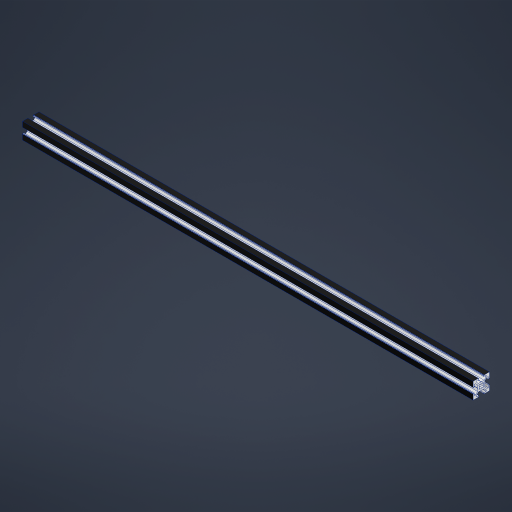
# Autodesk Inventor part: 20mm Extrusion 500mm
Saved by Autodesk Inventor 2024.2 (Build 282272000, 272)
## iProperties
Created: 2024-10-04
Part Number: 20mm Extrusion 500mm
Material: Aluminum 6061
Document SubType Name: Modeling
Designer: jerem
Density: 2.7 g/cm^3
Appearance: Aluminum - Flat
Author: jerem
Autodesk Inventor part; units mm, degrees
ref_plane "YZ Plane" through (0, 0, 0) normal (1, 0, 0) x (0, 1, 0)
ref_plane "XZ Plane" through (0, 0, 0) normal (0, 1, 0) x (-1, 0, 0)
ref_plane "XY Plane" through (0, 0, 0) normal (0, 0, 1) x (1, 0, 0)
sketch "Sketch1" plane through (0, 0, 0) normal (1, 0, 0) x (0, 1, 0)
  line L0 (-10, -10) -> (10, 10) construction
  line L1 (10, 10) -> (10, 3.5)
  line L2 (10, 3.5) -> (9.5, 3.5)
  line L3 (9.5, 3.5) -> (9.5, 3)
  line L4 (9.5, 3) -> (8.5, 3)
  line L5 (8.5, 3) -> (8.5, 5.95)
  line L6 (8.5, 5.95) -> (7.0107, 5.95)
  line L7 (7.0107, 5.95) -> (4.5, 3.4393)
  line L8 (4.5, 3.4393) -> (4.5, 0.1525)
  line L9 (2.4501, 2.4501) -> (3.0123, 1.888)
  line L10 (3.0123, 1.888) -> (2.4163, 1.292)
  arc A0 (2.74, 0) -> (2.4163, 1.292) centre (0, 0) ccw
  arc A1 (4.5, 0.1525) -> (4.3475, 0) centre (4.5, 0) ccw
  line L11 (10, 10) -> (2.4501, 2.4501)
  line L12 (4.3475, 0) -> (2.74, 0)
  line L13 (0, 0) -> (2.74, 0) construction
  line L14 (10, 10) -> (3.5, 10)
  line L15 (3.5, 10) -> (3.5, 9.5)
  line L16 (3.5, 9.5) -> (3, 9.5)
  line L17 (3, 9.5) -> (3, 8.5)
  line L18 (3, 8.5) -> (5.95, 8.5)
  line L19 (5.95, 8.5) -> (5.95, 7.0107)
  line L20 (5.95, 7.0107) -> (3.4393, 4.5)
  line L21 (3.4393, 4.5) -> (0.1525, 4.5)
  line L22 (2.4501, 2.4501) -> (1.888, 3.0123)
  line L23 (1.888, 3.0123) -> (1.292, 2.4163)
  arc A2 (1.292, 2.4163) -> (0, 2.74) centre (0, 0) ccw
  arc A3 (0, 4.3475) -> (0.1525, 4.5) centre (0, 4.5) ccw
  line L24 (0, 4.3475) -> (0, 2.74)
  line L25 (0, 0) -> (0, 2.74) construction
  line L26 (-8.5, 5.95) -> (-7.0107, 5.95)
  line L27 (-10, 3.5) -> (-9.5, 3.5)
  line L28 (-8.5, 3) -> (-8.5, 5.95)
  line L29 (-9.5, 3.5) -> (-9.5, 3)
  line L30 (-9.5, 3) -> (-8.5, 3)
  line L31 (-5.95, 8.5) -> (-5.95, 7.0107)
  line L32 (-7.0107, 5.95) -> (-4.5, 3.4393)
  line L33 (-5.95, 7.0107) -> (-3.4393, 4.5)
  line L34 (-10, 10) -> (-10, 3.5)
  line L35 (-10, 10) -> (-3.5, 10)
  line L36 (-10, 10) -> (-2.4501, 2.4501)
  line L37 (-3, 8.5) -> (-5.95, 8.5)
  line L38 (-3, 9.5) -> (-3, 8.5)
  line L39 (-3.5, 10) -> (-3.5, 9.5)
  line L40 (-3.5, 9.5) -> (-3, 9.5)
  line L41 (-3.4393, 4.5) -> (-0.1525, 4.5)
  line L42 (-2.4501, 2.4501) -> (-1.888, 3.0123)
  line L43 (-1.888, 3.0123) -> (-1.292, 2.4163)
  arc A4 (0, 2.74) -> (-1.292, 2.4163) centre (0, 0) ccw
  arc A5 (-0.1525, 4.5) -> (0, 4.3475) centre (0, 4.5) ccw
  line L44 (-2.4501, 2.4501) -> (-3.0123, 1.888)
  line L45 (-4.5, 3.4393) -> (-4.5, 0.1525)
  arc A6 (-4.3475, 0) -> (-4.5, 0.1525) centre (-4.5, 0) ccw
  line L46 (0, 4.3475) -> (0, 2.74)
  line L47 (-4.3475, 0) -> (-2.74, 0)
  arc A7 (-2.4163, 1.292) -> (-2.74, 0) centre (0, 0) ccw
  line L48 (0, 0) -> (0, 2.74) construction
  line L49 (-3.0123, 1.888) -> (-2.4163, 1.292)
  line L50 (-5.95, -8.5) -> (-5.95, -7.0107)
  line L51 (-3.5, -10) -> (-3.5, -9.5)
  line L52 (-3, -8.5) -> (-5.95, -8.5)
  line L53 (-3.5, -9.5) -> (-3, -9.5)
  line L54 (-3, -9.5) -> (-3, -8.5)
  line L55 (-8.5, -5.95) -> (-7.0107, -5.95)
  line L56 (-5.95, -7.0107) -> (-3.4393, -4.5)
  line L57 (-7.0107, -5.95) -> (-4.5, -3.4393)
  line L58 (-10, -10) -> (-3.5, -10)
  line L59 (-10, -10) -> (-10, -3.5)
  line L60 (-10, -10) -> (-2.4501, -2.4501)
  line L61 (-8.5, -3) -> (-8.5, -5.95)
  line L62 (-9.5, -3) -> (-8.5, -3)
  line L63 (-10, -3.5) -> (-9.5, -3.5)
  line L64 (-9.5, -3.5) -> (-9.5, -3)
  line L65 (-4.5, -3.4393) -> (-4.5, -0.1525)
  line L66 (-2.4501, -2.4501) -> (-3.0123, -1.888)
  line L67 (-3.0123, -1.888) -> (-2.4163, -1.292)
  arc A8 (-2.74, 0) -> (-2.4163, -1.292) centre (0, 0) ccw
  arc A9 (-4.5, -0.1525) -> (-4.3475, 0) centre (-4.5, 0) ccw
  line L68 (-2.4501, -2.4501) -> (-1.888, -3.0123)
  line L69 (-3.4393, -4.5) -> (-0.1525, -4.5)
  arc A10 (0, -4.3475) -> (-0.1525, -4.5) centre (0, -4.5) ccw
  line L70 (-4.3475, 0) -> (-2.74, 0)
  line L71 (0, -4.3475) -> (0, -2.74)
  arc A11 (-1.292, -2.4163) -> (0, -2.74) centre (0, 0) ccw
  line L72 (0, 0) -> (-2.74, 0) construction
  line L73 (-1.888, -3.0123) -> (-1.292, -2.4163)
  line L74 (8.5, -5.95) -> (7.0107, -5.95)
  line L75 (10, -3.5) -> (9.5, -3.5)
  line L76 (8.5, -3) -> (8.5, -5.95)
  line L77 (9.5, -3.5) -> (9.5, -3)
  line L78 (9.5, -3) -> (8.5, -3)
  line L79 (5.95, -8.5) -> (5.95, -7.0107)
  line L80 (7.0107, -5.95) -> (4.5, -3.4393)
  line L81 (5.95, -7.0107) -> (3.4393, -4.5)
  line L82 (10, -10) -> (10, -3.5)
  line L83 (10, -10) -> (3.5, -10)
  line L84 (10, -10) -> (2.4501, -2.4501)
  line L85 (3, -8.5) -> (5.95, -8.5)
  line L86 (3, -9.5) -> (3, -8.5)
  line L87 (3.5, -10) -> (3.5, -9.5)
  line L88 (3.5, -9.5) -> (3, -9.5)
  line L89 (3.4393, -4.5) -> (0.1525, -4.5)
  line L90 (2.4501, -2.4501) -> (1.888, -3.0123)
  line L91 (1.888, -3.0123) -> (1.292, -2.4163)
  arc A12 (0, -2.74) -> (1.292, -2.4163) centre (0, 0) ccw
  arc A13 (0.1525, -4.5) -> (0, -4.3475) centre (0, -4.5) ccw
  line L92 (2.4501, -2.4501) -> (3.0123, -1.888)
  line L93 (4.5, -3.4393) -> (4.5, -0.1525)
  arc A14 (4.3475, 0) -> (4.5, -0.1525) centre (4.5, 0) ccw
  line L94 (0, -4.3475) -> (0, -2.74)
  line L95 (4.3475, 0) -> (2.74, 0)
  arc A15 (2.4163, -1.292) -> (2.74, 0) centre (0, 0) ccw
  line L96 (0, 0) -> (0, -2.74) construction
  line L97 (3.0123, -1.888) -> (2.4163, -1.292)
  point P0 (9, 3)
  point P1 (3, 9)
  point P2 (-9, 3)
  point P3 (-3, 9)
  point P4 (-3, -9)
  point P5 (-9, -3)
  point P6 (9, -3)
  point P7 (3, -9)
  dimension "d2" = 6.5
  dimension "d3" = 0.5
  dimension "d4" = 4
  dimension "d5" = 3.465
  dimension "d6" = 5.48
  dimension "d7" = 0.795
  dimension "d8" = 0.305
  dimension "d9" = 2.95
  dimension "d11" = 0.75
  dimension "d14" = 45
  dimension "d15" = 10
  dimension "d16" = 1
  dimension "d17" = 3
  dimension "d18" = 45
  dimension "d21" = 360
  constraints: 196 end point, 32 point on circle, 16 centre point, 14 symmetric about line, 6 perpendicular, 3 coincident, 3 horizontal, 2 line through centre, 2 midpoint, 2 parallel, 1 collinear, 1 point on line, 237 other
  measures "d2" distance of L0.end L1.end
  measures "d3" distance from line of L1.end L3
  measures "d4" distance between parallel lines of L8 L5
  measures "d5" distance from line of point (0, 0) L9
  measures "d6" diameter of A0
  measures "d7" distance from line of L11 L9.end
  measures "d8" diameter of A1
  measures "d9" distance of L4.end L5.end
  measures "d11" distance between parallel lines of L0 L7
  measures "d14" angle of L1 L11
  measures "d15" distance from line of point (0, 0) L1
  measures "d16" distance of L3.end L4.end
  measures "d17" distance between parallel lines of L12 L4
  measures "d18" angle of L0 L12
extrude "Extrusion1" add sketch "Sketch1" along normal blind 550 contours L1 L2 L3 L4 L5 L6 L7 L8 A1 L12 A0 L10 L9 L11 | L11 L22 L23 A2 L24 A3 L21 L20 L19 L18 L17 L16 L15 L14 | L12 A14 L93 L80 L74 L76 L78 L77 L75 L82 L84 L92 L97 A15 | A4 L43 L42 L36 L35 L39 L40 L38 L37 L31 L33 L41 A5 L24 | L84 L83 L87 L88 L86 L85 L79 L81 L89 A13 L71 A12 L91 L90 | L44 L49 A7 L47 A6 L45 L32 L26 L28 L30 L29 L27 L34 L36 | L71 A10 L69 L56 L50 L52 L54 L53 L51 L58 L60 L68 L73 A11 | A8 L67 L66 L60 L59 L63 L64 L62 L61 L55 L57 L65 A9 L47
body "Solid1"
